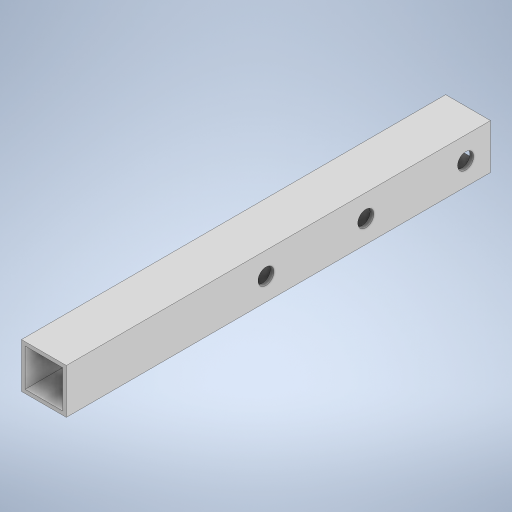
# Autodesk Inventor part: squareEx1
Saved by Autodesk Inventor 2023 (Build 270158000, 158)
## iProperties
Created: 2022-12-04
Part Number: squareEx1
Material: 一般
Document SubType Name: Modeling
Designer: RiSA
Density: 1 g/cm^3
Appearance: 既定
Author: RiSA
Autodesk Inventor part; units mm, degrees
ref_plane "YZ Plane" through (0, 0, 0) normal (1, 0, 0) x (0, 1, 0)
ref_plane "XZ Plane" through (0, 0, 0) normal (0, 1, 0) x (-1, 0, 0)
ref_plane "XY Plane" through (0, 0, 0) normal (0, 0, 1) x (1, 0, 0)
sketch "スケッチ1" plane through (0, 0, 0) normal (0, 0, 1) x (1, 0, 0)
  line L0 (4.5, -4.5) -> (-4.5, -4.5)
  line L1 (-4.5, -4.5) -> (-4.5, 4.5)
  line L2 (-4.5, 4.5) -> (4.5, 4.5)
  line L3 (4.5, 4.5) -> (4.5, -4.5)
  line L4 (4.5, -4.5) -> (-4.5, 4.5) construction
  line L5 (-4.5, -4.5) -> (4.5, 4.5) construction
  line L6 (3.75, -3.75) -> (-3.75, -3.75)
  line L7 (-3.75, -3.75) -> (-3.75, 3.75)
  line L8 (-3.75, 3.75) -> (3.75, 3.75)
  line L9 (3.75, 3.75) -> (3.75, -3.75)
  line L10 (3.75, -3.75) -> (-3.75, 3.75) construction
  line L11 (-3.75, -3.75) -> (3.75, 3.75) construction
  point P0 (0, 0)
  dimension "d0" = 9
  dimension "d1" = 9
  dimension "d2" = 7.5
  dimension "d3" = 7.5
  constraints: 24 end point, 4 midpoint, 4 parallel, 2 horizontal, 2 perpendicular
  measures "d0" distance of L1.end L2.end
  measures "d1" distance of L0.end L1.end
  measures "d2" distance of L7.end L8.end
  measures "d3" distance of L6.end L7.end
extrude "押し出し1" add sketch "スケッチ1" along normal blind 90
sketch "スケッチ2" plane through (4.5, -4.5, 0) normal (1, 0, 0) x (0, 0, -1)
  line L0 (0, 0) -> (-90, 0) projected
  line L1 (0, 0) -> (0, 9) projected
  point P0 (0, 4.5)
  point P1 (-5, 4.5)
  point P2 (-25, 4.5)
  point P3 (-45, 4.5)
  dimension "d6" = 4.5
  dimension "d7" = 5
  dimension "d8" = 20
  dimension "d9" = 20
  measures "d6" distance from line of L0 point (-5, 4.5)
  measures "d7" distance from line of L1 point (-5, 4.5)
  measures "d8" distance of point (-5, 4.5) point (-25, 4.5)
  measures "d9" distance of point (-25, 4.5) point (-45, 4.5)
hole "穴1" at (4.5, 0, 5) at (4.5, 0, 25) at (4.5, 0, 45) direction (-1, 0, 0) diameter 3.2 end through all
sketch "スケッチ3" plane through (0, 0, 90) normal (0, 0, 1) x (1, 0, 0)
  line L0 (4.5, -4.5) -> (-4.5, -4.5)
  line L1 (-4.5, -4.5) -> (-4.5, 4.5)
  line L2 (-4.5, 4.5) -> (4.5, 4.5)
  line L3 (4.5, 4.5) -> (4.5, -4.5)
  line L4 (4.5, -4.5) -> (-4.5, 4.5) construction
  line L5 (-4.5, -4.5) -> (4.5, 4.5) construction
  point P0 (0, 0)
  constraints: 12 end point, 2 midpoint, 2 parallel, 1 horizontal, 1 perpendicular
extrude "押し出し2" cut sketch "スケッチ3" against normal blind 5
